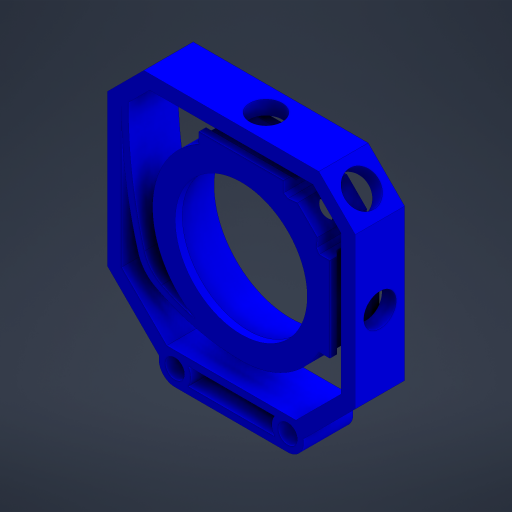
# Autodesk Inventor part: One Inch Lense Holder (V5)
Saved by Autodesk Inventor 2023.4 (Build 274418000, 418)
## iProperties
Created: 2022-07-25
Part Number: One Inch Lense Holder (V5)
Material: Generic
Document SubType Name: Modeling
Designer: xSibe
Density: 1 g/cm^3
Appearance: Plastic Blue
Author: xSibe
Autodesk Inventor part; units mm, degrees
ref_plane "YZ Plane" through (0, 0, 0) normal (1, 0, 0) x (0, 1, 0)
ref_plane "XZ Plane" through (0, 0, 0) normal (0, 1, 0) x (-1, 0, 0)
sketch "Sketch1" plane through (0, 0, 0) normal (0, 0, 1) x (1, 0, 0)
  circle A0 centre (10, 3.85) radius 1.5625
  circle A1 centre (-10, 3.85) radius 1.5625
  line L0 (-16.9, 0) -> (16.9, 0)
  line L1 (16.9, 0) -> (16.9, 7.7)
  line L2 (-16.9, 7.7) -> (16.9, 7.7)
  line L3 (-16.9, 0) -> (-16.9, 7.7)
  circle A2 centre (-10, 3.85) radius 2.8125
  circle A3 centre (10, 3.85) radius 2.8125
  line L4 (-10, 6.6625) -> (10, 6.6625)
  line L5 (10, 1.0375) -> (-10, 1.0375)
  line L6 (-10, 2.2875) -> (10, 2.2875)
  line L7 (-10, 5.4125) -> (10, 5.4125)
  line L8 (-17.05, 7.7) -> (-17.05, 42.1)
  line L9 (17.05, 7.7) -> (17.05, 42.1)
  line L10 (-17.05, 24.9) -> (17.05, 24.9)
  line L11 (0, 24.9) -> (1.767767, 26.667767)
  line L12 (0, 24.9) -> (2.5, 24.9) construction
  circle A4 centre (1.767767, 26.667767) radius 13.575
  circle A5 centre (1.767767, 26.667767) radius 11.075
  circle A6 centre (1.767767, 26.667767) radius 15.7
  line L13 (1.767767, 26.667767) -> (1.767767, 42.367767)
  line L14 (1.767767, 42.367767) -> (1.767767, 41.367767)
  line L15 (-5.732233, 40.367767) -> (9.267767, 40.367767)
  line L16 (9.267767, 40.367767) -> (9.267767, 42.367767)
  line L17 (9.267767, 42.367767) -> (-5.732233, 42.367767)
  line L18 (-5.732233, 42.367767) -> (-5.732233, 40.367767)
  line L19 (-5.732233, 40.367767) -> (9.267767, 42.367767) construction
  line L20 (9.267767, 40.367767) -> (-5.732233, 42.367767) construction
  line L21 (1.767767, 26.667767) -> (12.869343, 37.769343)
  line L22 (12.869343, 37.769343) -> (12.427402, 37.327402)
  line L23 (15.255829, 36.620295) -> (11.720295, 40.155829)
  line L24 (11.720295, 40.155829) -> (9.598975, 38.034508)
  line L25 (9.598975, 38.034508) -> (13.134508, 34.498975)
  line L26 (13.134508, 34.498975) -> (15.255829, 36.620295)
  line L27 (15.255829, 36.620295) -> (9.598975, 38.034508) construction
  line L28 (11.720295, 40.155829) -> (13.134508, 34.498975) construction
  line L29 (15.255829, 36.620295) -> (20.255829, 36.620295) construction
  line L30 (15.467767, 19.167767) -> (15.467767, 34.167767)
  line L31 (15.467767, 34.167767) -> (17.467767, 34.167767)
  line L32 (17.467767, 34.167767) -> (17.467767, 19.167767)
  line L33 (17.467767, 19.167767) -> (15.467767, 19.167767)
  line L34 (1.767767, 42.367767) -> (1.767767, 44.367767)
  line L35 (17.467767, 26.667767) -> (19.467767, 26.667767)
  line L36 (-10.217767, 5.432233) -> (10.217767, 5.432233)
  line L37 (19.467767, 14.682233) -> (19.467767, 39.367767)
  line L38 (14.467767, 44.367767) -> (-14.467767, 44.367767)
  line L39 (-19.467767, 39.367767) -> (-19.467767, 14.682233)
  line L40 (-19.467767, 5.432233) -> (19.467767, 44.367767) construction
  line L41 (19.467767, 5.432233) -> (-19.467767, 44.367767) construction
  line L42 (-10.217767, 5.432233) -> (-19.467767, 14.682233)
  line L43 (10.217767, 5.432233) -> (19.467767, 14.682233)
  line L44 (14.467767, 44.367767) -> (19.467767, 39.367767)
  line L45 (-14.467767, 44.367767) -> (-19.467767, 39.367767)
  line L46 (-15.503301, 46.867767) -> (-21.967767, 40.403301)
  line L47 (-21.967767, 40.403301) -> (-21.967767, 13.646699)
  line L48 (-21.967767, 13.646699) -> (-11.253301, 2.932233)
  line L49 (-11.253301, 2.932233) -> (11.253301, 2.932233)
  line L50 (11.253301, 2.932233) -> (21.967767, 13.646699)
  line L51 (21.967767, 13.646699) -> (21.967767, 40.403301)
  line L52 (21.967767, 40.403301) -> (15.503301, 46.867767)
  line L53 (15.503301, 46.867767) -> (-15.503301, 46.867767)
  circle A7 centre (-10, 3.85) radius 1.705
  circle A8 centre (10, 3.85) radius 1.707
  line L54 (1.767767, 10.967767) -> (-15.732233, 10.967767)
  arc A9 (-15.732233, 15.967767) -> (1.767767, 10.967767) centre (1.767767, 44.092767) ccw
  line L55 (-15.732233, 10.967767) -> (-15.732233, 15.967767)
  arc A10 (-19.467767, 39.367767) -> (-15.732233, 15.967767) centre (55.690728, 39.367767) ccw
  arc A11 (-18.207013, 40.628521) -> (-14.685576, 16.792526) centre (55.690728, 39.367767) ccw
  arc A12 (-14.685576, 16.792526) -> (-6.464552, 13.299187) centre (1.767767, 44.092767) ccw
  arc A13 (-16.470968, 18.356128) -> (-13.426005, 14.65784) centre (-10.64074, 20.053742) ccw
  line L56 (-15.732233, 15.967767) -> (-16.470968, 18.356128)
  line L57 (-14.685576, 16.792526) -> (-15.408827, 19.185622)
  arc A14 (-15.408827, 19.185622) -> (-12.355566, 15.517479) centre (-9.748456, 20.792361) ccw
  line L58 (-10, 6.6625) -> (-11.448034, 6.6625)
  line L59 (10, 6.6625) -> (11.448034, 6.6625)
  point P0 (0, 0)
  point P1 (-18.192161, 40.643373)
  point P2 (-7.661464, 2.2875)
  point P3 (-7.661464, 5.4125)
  point P4 (7.661464, 5.4125)
  point P5 (7.661464, 2.2875)
  point P6 (7.341455, 2.932233)
  point P7 (-7.341455, 2.932233)
  point P8 (-11.185824, 6.40029)
  point P9 (11.185824, 6.40029)
  point P10 (-5.732233, 40.460519)
  point P11 (15.560519, 19.167767)
  point P12 (15.560519, 34.167767)
  point P13 (14.495461, 35.859927)
  point P14 (10.959927, 39.395461)
  point P15 (9.267767, 40.460519)
  point P16 (12.751875, 4.430808)
  point P17 (-12.751875, 4.430808)
  point P18 (-7.831162, 14.243977)
  point P19 (7.67477, 5.432233)
  point P20 (-7.67477, 5.432233)
  point P21 (-16.411283, 18.163163)
  point P22 (-15.351247, 18.995103)
  point P23 (-17.05, 20.457826)
  point P24 (-17.05, 26.281434)
  point P25 (-16.787885, 24.9)
  point P26 (-17.05, 12.264466)
  point P27 (-17.05, 41.785534)
  dimension "d0" = 1.25
  dimension "d1" = 1.25
  dimension "d2" = 2.5
  dimension "d3" = 45
  dimension "d4" = 27.15
  dimension "d5" = 2.5
  dimension "d6" = 2.125
  dimension "d7" = 1
  dimension "d8" = 15
  dimension "d9" = 2
  dimension "d10" = 0.625
  dimension "d11" = 5
  dimension "d12" = 135
  dimension "d13" = 3
  dimension "d14" = 2
  dimension "d15" = 2
  dimension "d16" = 38.93553
  dimension "d17" = 38.93553
  dimension "d18" = 9.25
  dimension "d19" = 9.25
  dimension "d20" = 9.25
  dimension "d21" = 9.25
  dimension "d22" = 5
  dimension "d23" = 5
  dimension "d24" = 5
  dimension "d25" = 5
  dimension "d26" = 2.5
  dimension "d46" = 0.1425
  dimension "d47" = 0.1445
  dimension "d48" = 17.5
  dimension "d49" = 5
  dimension "d50" = 1.25
  dimension "d51" = 2.5
  dimension "d52" = 2.5
  constraints: 108 end point, 28 point on circle, 16 point on line, 15 tangent, 13 centre point, 10 midpoint, 8 horizontal, 8 parallel, 6 perpendicular, 4 symmetric about line, 2 equal length, 2 vertical, 1 coincident, 8 other
  measures "d0" radial gap between concentric circles of A1 A2
  measures "d1" radial gap between concentric circles of A0 A3
  measures "d2" distance of L11.start L11.end
  measures "d3" angle of L12 L11
  measures "d4" diameter of A4
  measures "d5" radial gap between concentric circles of A4 A5
  measures "d6" radial gap between concentric circles of A4 A6
  measures "d7" distance of L13.end L14.end
  measures "d8" distance of L17.end L16.end
  measures "d9" distance of L16.end L15.end
  measures "d10" distance of L21.end L22.end
  measures "d11" distance of L23.start L23.end
  measures "d12" angle of L29 L23
  measures "d13" distance of L24.end L23.end
  measures "d14" distance of L13.end L34.end
  measures "d15" distance of L35.start L35.end
  measures "d16" distance of L40.end L41.end
  measures "d17" distance of L41.end L40.start
  measures "d18" distance of L36.start L40.start
  measures "d19" distance of L39.end L40.start
  measures "d20" distance of L36.end L41.start
  measures "d21" distance of L37.start L41.start
  measures "d22" distance of L38.start L40.end
  measures "d23" distance of L37.end L40.end
  measures "d24" distance of L38.end L41.end
  measures "d25" distance of L39.start L41.end
  measures "d26" distance between parallel lines of L38 L53
  measures "d46" radial gap between concentric circles of A1 A7
  measures "d47" radial gap between concentric circles of A0 A8
  measures "d48" distance of L54.start L54.end
  measures "d49" distance of L54.end L55.end
  measures "d50" radial gap between concentric circles of A10 A11
  measures "d51" distance of L55.end L56.end
  measures "d52" distance of L57.start L57.end
sketch "Sketch1 outline for Extrusion1" plane through (0, 0, 0) normal (0, 0, 1) x (1, 0, 0)
  line L0 (-7.661464, 5.4125) -> (7.661464, 5.4125)
  arc A0 (7.661464, 5.4125) -> (7.661464, 2.2875) centre (10, 3.85) ccw
  line L1 (7.661464, 2.2875) -> (-7.661464, 2.2875)
  arc A1 (-7.661464, 2.2875) -> (-7.661464, 5.4125) centre (-10, 3.85) ccw
  arc A2 (10, 1.0375) -> (12.751875, 4.430808) centre (10, 3.85) ccw
  line L2 (12.751875, 4.430808) -> (21.967767, 13.646699)
  line L3 (21.967767, 13.646699) -> (21.967767, 40.403301)
  line L4 (21.967767, 40.403301) -> (15.503301, 46.867767)
  line L5 (15.503301, 46.867767) -> (-15.503301, 46.867767)
  line L6 (-15.503301, 46.867767) -> (-21.967767, 40.403301)
  line L7 (-21.967767, 40.403301) -> (-21.967767, 13.646699)
  line L8 (-21.967767, 13.646699) -> (-12.751875, 4.430808)
  arc A3 (-12.751875, 4.430808) -> (-10, 1.0375) centre (-10, 3.85) ccw
  line L9 (-10, 1.0375) -> (10, 1.0375)
  circle A4 centre (1.767767, 26.667767) radius 13.575
  line L10 (-11.448034, 6.6625) -> (-19.467767, 14.682233)
  line L11 (-19.467767, 14.682233) -> (-19.467767, 39.367767)
  arc A5 (-19.467767, 39.367767) -> (-16.470968, 18.356128) centre (55.690728, 39.367767) ccw
  arc A6 (-16.470968, 18.356128) -> (-13.426005, 14.65784) centre (-10.64074, 20.053742) ccw
  arc A7 (-13.426005, 14.65784) -> (1.767767, 10.967767) centre (1.767767, 44.092767) ccw
  arc A8 (1.767767, 10.967767) -> (15.560519, 19.167767) centre (1.767767, 26.667767) ccw
  line L12 (15.560519, 19.167767) -> (17.467767, 19.167767)
  line L13 (17.467767, 19.167767) -> (17.467767, 34.167767)
  line L14 (17.467767, 34.167767) -> (15.560519, 34.167767)
  arc A9 (15.560519, 34.167767) -> (14.495461, 35.859927) centre (1.767767, 26.667767) ccw
  line L15 (14.495461, 35.859927) -> (15.255829, 36.620295)
  line L16 (15.255829, 36.620295) -> (11.720295, 40.155829)
  line L17 (11.720295, 40.155829) -> (10.959927, 39.395461)
  arc A10 (10.959927, 39.395461) -> (9.267767, 40.460519) centre (1.767767, 26.667767) ccw
  line L18 (9.267767, 40.460519) -> (9.267767, 42.367767)
  line L19 (9.267767, 42.367767) -> (-5.732233, 42.367767)
  line L20 (-5.732233, 42.367767) -> (-5.732233, 40.460519)
  arc A11 (-5.732233, 40.460519) -> (-6.464552, 13.299187) centre (1.767767, 26.667767) ccw
  arc A12 (-6.464552, 13.299187) -> (-12.355566, 15.517479) centre (1.767767, 44.092767) cw
  arc A13 (-12.355566, 15.517479) -> (-15.408827, 19.185622) centre (-9.748456, 20.792361) cw
  arc A14 (-15.408827, 19.185622) -> (-18.207013, 40.628521) centre (55.690728, 39.367767) cw
  line L21 (-18.207013, 40.628521) -> (-14.467767, 44.367767)
  line L22 (-14.467767, 44.367767) -> (14.467767, 44.367767)
  line L23 (14.467767, 44.367767) -> (19.467767, 39.367767)
  line L24 (19.467767, 39.367767) -> (19.467767, 14.682233)
  line L25 (19.467767, 14.682233) -> (11.448034, 6.6625)
  line L26 (11.448034, 6.6625) -> (-11.448034, 6.6625)
  circle A15 centre (-10, 3.85) radius 1.705
  circle A16 centre (10, 3.85) radius 1.707
extrude "Extrusion1" add sketch "Sketch1 outline for Extrusion1" along normal mid plane 8.75
sketch "Sketch2" plane through (0, 0, 0) normal (0, 0, 1) x (1, 0, 0)
  circle A0 centre (1.767767, 26.667767) radius 13.575
  circle A1 centre (1.767767, 26.667767) radius 11.7
  point P0 (0, 0)
  dimension "d30" = 1.875
  constraints: 1 centre point
  measures "d30" radial gap between concentric circles of A0 A1
sketch "Sketch2 outline for Extrusion2" plane through (0, 0, 0) normal (0, 0, 1) x (1, 0, 0)
  circle A0 centre (1.767767, 26.667767) radius 13.575
  circle A1 centre (1.767767, 26.667767) radius 11.7
extrude "Extrusion2" add sketch "Sketch2 outline for Extrusion2" against normal blind 1.25 from surface at 4.375
sketch "Sketch3" plane through (21.967767, 13.646699, -4.375) normal (1, 0, 0) x (0, 0, -1)
  line L0 (0, 5.521068) -> (-8.75, 5.521068)
  line L1 (0, 20.521068) -> (0, 5.521068)
  line L2 (0, 20.521068) -> (-8.75, 20.521068)
  line L3 (-8.75, 5.521068) -> (-8.75, 20.521068)
  line L4 (-4.375, 20.521068) -> (-4.375, 5.521068)
  circle A0 centre (-4.375, 13.021068) radius 2.875
  point P0 (-4.375, -13.646699)
  dimension "d33" = 5.75
  constraints: 3 midpoint, 2 end point, 1 centre point
  measures "d33" diameter of A0
sketch "Sketch3 outline for Extrusion3" plane through (21.967767, 13.646699, -4.375) normal (1, 0, 0) x (0, 0, -1)
  circle A0 centre (-4.375, 13.021068) radius 2.875
extrude "Extrusion3" cut sketch "Sketch3 outline for Extrusion3" against normal up to surface (2.5 mm away)
sketch "Sketch4" plane through (15.560519, 34.167767, -4.375) normal (0, 1, 0) x (1, 0, 0)
  line L0 (1.907248, 0) -> (1.907248, -8.75)
  line L1 (0, 0) -> (1.907248, 0)
  line L2 (0, 0) -> (0, -8.75)
  line L3 (1.907248, -8.75) -> (0, -8.75)
  line L4 (1.907248, -8.75) -> (0, -8.75)
  line L5 (0, -8.75) -> (0, -7.5)
  line L6 (0, -7.5) -> (1.907248, -7.5)
  line L7 (1.907248, -7.5) -> (1.907248, -8.75)
  line L8 (1.907248, -7.5) -> (0, -5.592752)
  line L9 (1.907248, -7.5) -> (4.604505, -7.5) construction
  line L10 (0, -4.375) -> (1.907248, -4.375)
  line L11 (1.907248, -1.25) -> (0, -3.157248)
  line L12 (0.953624, -8.75) -> (0.953624, 0)
  point P0 (-15.560519, -4.375)
  point P1 (1.907248, -1.25)
  point P2 (0, -3.157248)
  point P3 (1.907248, -7.5)
  point P4 (0.953624, -2.203624)
  point P5 (0.953624, -6.546376)
  dimension "d36" = 1.25
  dimension "d37" = 135
  constraints: 18 end point, 4 midpoint, 2 horizontal, 2 parallel, 2 point on line, 2 symmetric about line, 1 equal length, 1 perpendicular
  measures "d36" distance of L4.end L5.end
  measures "d37" angle of L9 L8
sketch "Sketch4 outline for Extrusion4" plane through (15.560519, 34.167767, -4.375) normal (0, 1, 0) x (1, 0, 0)
  line L0 (0.953624, -2.203624) -> (0.953624, -6.546376)
  line L1 (1.907248, -1.25) -> (0.953624, -2.203624)
  line L2 (1.907248, -7.5) -> (1.907248, -1.25)
  line L3 (0.953624, -6.546376) -> (1.907248, -7.5)
extrude "Extrusion4" cut sketch "Sketch4 outline for Extrusion4" against normal up to surface (15 mm away)
ref_plane "Work Plane1" through (17.467767, 42.367767, 4.375) normal (0.7071068, -0.7071068, 0) x (0, 0, -1)
mirror "Mirror1" about plane through (17.467767, 42.367767, 4.375) normal (0.7071068, -0.7071068, 0) of "Extrusion3", "Extrusion4"
sketch "Sketch5" plane through (21.967767, 40.403301, 4.375) normal (0.7071068, 0.7071068, 0) x (0.7071068, -0.7071068, 0)
  line L0 (0, 8.75) -> (0, 0)
  line L1 (-9.142136, 8.75) -> (0, 8.75)
  line L2 (-9.142136, 8.75) -> (-9.142136, 0)
  line L3 (0, 0) -> (-9.142136, 0)
  line L4 (-2.071068, 8.75) -> (-2.071068, 0)
  line L5 (-7.071068, 8.75) -> (-2.071068, 8.75)
  line L6 (-7.071068, 8.75) -> (-7.071068, 0)
  line L7 (-2.071068, 0) -> (-7.071068, 0)
  circle A0 centre (-4.571068, 4.375) radius 1.875
  line L8 (-7.071068, 4.375) -> (-2.071068, 4.375)
  circle A1 centre (-4.571068, 4.375) radius 3
  point P0 (13.035891, 4.375)
  dimension "d40" = 3.75
  dimension "d41" = 6
  constraints: 3 midpoint, 2 centre point, 2 end point, 1 coincident
  measures "d40" diameter of A0
  measures "d41" diameter of A1
sketch "Sketch5 outline for Extrusion5" plane through (21.967767, 40.403301, 4.375) normal (0.7071068, 0.7071068, 0) x (0.7071068, -0.7071068, 0)
  circle A0 centre (-4.571068, 4.375) radius 3
extrude "Extrusion5" cut sketch "Sketch5 outline for Extrusion5" against normal up to surface (2.5 mm away)
sketch "Sketch5 outline for Extrusion6" plane through (21.967767, 40.403301, 4.375) normal (0.7071068, 0.7071068, 0) x (0.7071068, -0.7071068, 0)
  circle A0 centre (-4.571068, 4.375) radius 1.875
extrude "Extrusion6" cut sketch "Sketch5 outline for Extrusion6" against normal up to next from surface at -7.421046
chamfer "Chamfer1" distance 1.075 angle 45 2 edges at (14.4955, 35.8599, 0) (10.9599, 39.3955, 0)
equation "\"d19\" = d18"
equation "\"d20\" = d18"
equation "\"d21\" = d20"
equation "\"d23\" = d22"
equation "\"d24\" = d22"
equation "\"d25\" = d24"
body "Solid1"
